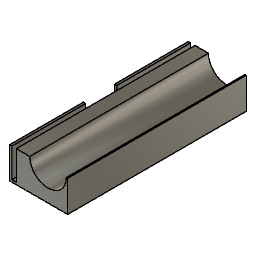
Straw Mount Slot V1 (Autodesk Fusion 360 design; units mm, degrees)
Autodesk Fusion 360 part; units mm, degrees
sketch "Sketch1" plane through (0, 0, 0) normal (0, 0, 1) x (1, 0, 0)
  line L0 (0, 0) -> (13, 0)
  line L1 (13, 0) -> (13, 40)
  line L2 (13, 40) -> (0, 40)
  line L3 (0, 40) -> (0, 0)
  dimension "d1" = 13
  dimension "d2" = 40
  constraint horizontal L0
  constraint vertical L1
  constraint horizontal L2
  constraint vertical L3
  constraint coincident L0.start L3.end
  measures "d1" distance of L0.start L0.end
  measures "d2" distance of L0.start L2.end
extrude "Extrude1" add sketch "Sketch1" along normal blind 7 and the other way blind 0
sketch "Sketch2" plane through (0, 0, 0) normal (0, -1, 0) x (1, 0, 0)
  line L0 (0, 0) -> (13, 0)
  line L1 (13, 0) -> (13, 7)
  line L2 (13, 7) -> (0, 7)
  line L3 (0, 7) -> (0, 0)
  circle A0 centre (8.6106, 7) radius 4.1
  dimension "d5" = 8.2
  constraint coincident L2 A0.centre
  measures "d5" diameter of A0
extrude "Extrude2" cut sketch "Sketch2" against normal blind 41 contours L2 A0 picked at (8.104, 4.6437)
sketch "Sketch4" plane through (0, 0, 7) normal (0, 0, 1) x (-1, 0, 0)
  line L0 (-4.5106, 0) -> (-4.5106, -40)
  line L1 (-4.5106, -40) -> (0, -40)
  line L2 (0, -40) -> (0, 0)
  line L3 (0, 0) -> (-4.5106, 0)
  line L4 (-0.517, -40) -> (-1.5, -40)
  line L5 (-1.5, -40) -> (-1.5, 0)
  line L6 (-1.5, 0) -> (-0.517, 0)
  line L7 (-0.517, 0) -> (-0.517, -40)
  constraint horizontal L4
  constraint vertical L5
  constraint horizontal L6
  constraint vertical L7
  constraint coincident L3 L5.end
  constraint coincident L1 L4.start
extrude "Extrude4" cut sketch "Sketch4" against normal blind 6.5 contours L1 L3 L4 L5 L6 L7
sketch "Sketch5" plane through (0, 0, 0) normal (-1, 0, 0) x (0, -1, 0)
  line L0 (-40, 0) -> (0, 0)
  line L1 (0, 0) -> (0, 7)
  line L2 (0, 7) -> (-40, 7)
  line L3 (-40, 7) -> (-40, 0)
  circle A0 centre (-20, 3.9772) radius 3.5
  line L4 (-23.5, 3.9917) -> (-23.4875, 7)
  line L5 (-16.5, 3.9917) -> (-16.5125, 7)
  dimension "d15" = 7
  constraint coincident A0 L4.start
  constraint coincident L2 L4.end
  constraint tangent A0 L4
  constraint coincident A0 L5.start
  constraint coincident L2 L5.end
  constraint tangent A0 L5
  measures "d15" diameter of A0
extrude "Extrude5" cut sketch "Sketch5" against normal blind 1 contours L2 A0 L4 | L2 A0 L5 | L2 A0 picked at (-20.0897, 4.8292)
